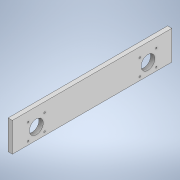
# Autodesk Inventor part: bok
Saved by Autodesk Inventor 2020 (Build 240168000, 168)
## iProperties
Created: 2020-03-28
Part Number: bok
Material: Ogólny
Document SubType Name: Modeling
Designer: niedz
Density: 1 g/cm^3
Appearance: Domyślna
Author: niedz
Autodesk Inventor part; units mm, degrees
ref_plane "YZ Plane" through (0, 0, 0) normal (1, 0, 0) x (0, 1, 0)
ref_plane "XZ Plane" through (0, 0, 0) normal (0, 1, 0) x (-1, 0, 0)
ref_plane "XY Plane" through (0, 0, 0) normal (0, 0, 1) x (1, 0, 0)
sketch "Szkic1" plane through (0, 0, 0) normal (1, 0, 0) x (0, 1, 0)
  line L0 (0, -300) -> (55, -300)
  line L1 (55, 0) -> (0, 0)
  line L2 (55, 0) -> (55, -300)
  circle A0 centre (22, -45) radius 13
  circle A1 centre (22, -255) radius 13
  line L3 (0, 0) -> (0, -300)
  circle A2 centre (37.5154, -29.5) radius 1.5
  circle A3 centre (6.5, -29.4846) radius 1.5
  circle A4 centre (6.4846, -60.5) radius 1.5
  circle A5 centre (37.5, -60.5154) radius 1.5
  circle A6 centre (6.5, -270.5) radius 1.5
  circle A7 centre (37.5, -270.5) radius 1.5
  circle A8 centre (37.5, -239.5) radius 1.5
  circle A9 centre (6.5, -239.5) radius 1.5
  dimension "d0" = 300
  dimension "d1" = 55
  dimension "d2" = 300
  dimension "d5" = 26
  dimension "d8" = 26
  dimension "d9" = 3
  dimension "d12" = 360
  dimension "d14" = 3
  dimension "d17" = 360
  constraints: 10 centre point, 8 end point, 2 vertical, 18 other
  measures "d0" distance of L1.end L0.start
  measures "d1" distance of L0.start L0.end
  measures "d2" distance of L0.end L1.start
  measures "d5" diameter of A0
  measures "d8" diameter of A1
  measures "d9" diameter of A2
  measures "d14" diameter of A6
extrude "Wyciągnięcie proste1" add sketch "Szkic1" along normal blind 8
